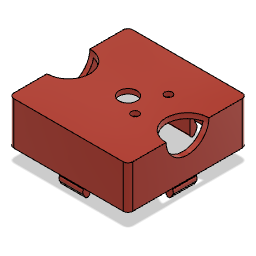
probatio_block_top_rotary_encoder_unthreaded_with_breakout_board_v2 (Autodesk Fusion 360 design; units mm, degrees)
Autodesk Fusion 360 part; units mm, degrees
note: some values were not read from the file. Chosen so that the rebuilt part matches the saved one: which face or edge a step refers to. Set by a fixed rule: which sketch regions a step uses.
ref_plane "WorkPlane1" through (0, 0, 56) normal (0, 0, 1) x (1, 0, 0)
sketch "top" plane through (0, 0, 56) normal (0, 0, 1) x (1, 0, 0)
  line L0 (25, -25) -> (-25, -25)
  line L1 (-25, -25) -> (-25, 25)
  line L2 (-25, 25) -> (25, 25)
  line L3 (25, 25) -> (25, -25)
  line L4 (25, -25) -> (-25, 25) construction
  line L5 (-25, -25) -> (25, 25) construction
  dimension "d12" = 50
  dimension "d13" = 50
  constraint perpendicular L0 L1
  constraint parallel L0 L2
  constraint parallel L1 L3
  constraint horizontal L0
  constraint coincident L4 origin
  constraint coincident L5 origin
  measures "d12" distance of L0.end L1.end
  measures "d13" distance of L1.end L2.end
extrude "Extrude1" add sketch "top" against normal blind 18 makes body 1
fillet "Fillet1" radius 2 4 edges at (-25, 25, 47) (25, 25, 47) (25, -25, 47) (-25, -25, 47) on bodies 1
shell "Shell1" thickness 2 removed faces 1 at (8.3333, -7.6667, 38) on bodies 1
sketch "handle" plane through (25, 0, 0) normal (1, 0, 0) x (0, 0, -1)
  line L0 (-38, -23) -> (-38, 23)
  line L1 (-56, 23) -> (-56, -23)
  line L2 (-56, 23) -> (-56, -23)
  circle A0 centre (-56, 0) radius 7
  line L3 (-56, -23) -> (-38, -23)
  line L4 (-38, 23) -> (-56, 23)
  line L5 (-38, 23) -> (-38, -23)
  circle A1 centre (-56, 0) radius 9
  dimension "d95" = 14
  dimension "d159" = 2
  constraint midpoint L1 A0.centre
  constraint concentric A0 A1
  measures "d95" diameter of A0
  measures "d159" distance of A0 A1
revolve "Revolve1" cut sketch "handle" angle 90 about axis through (25, 23, 56) along (0, 1, 0) contours L1 L2 A0 picked at (-50.399, -0.5675) bodies 1
revolve "Revolve2" cut sketch "handle" angle 90 about axis through (25, 23, 56) along (0, 1, 0) contours L1 L2 A0 A1 picked at (-54.0705, -8.0868) bodies 1
mirror "Mirror9" about plane through (0, 0, 0) normal (1, 0, 0) of "Revolve1", "Revolve2"
sketch "customisable" plane through (0, 0, 56) normal (0, 0, 1) x (1, 0, 0)
  line L0 (-25, -9) -> (-25, -23)
  line L1 (-23, -25) -> (23, -25)
  line L2 (23, 25) -> (-23, 25)
  line L3 (0.05, 0.05) -> (-0.05, 0.05)
  line L4 (-0.05, 0.05) -> (-0.05, -0.05)
  line L5 (-0.05, -0.05) -> (0.05, -0.05)
  line L6 (0.05, -0.05) -> (0.05, 0.05)
  line L7 (0.05, 0.05) -> (-0.05, -0.05) construction
  line L8 (-0.05, 0.05) -> (0.05, -0.05) construction
  arc A0 (-25, -23) -> (-23, -25) centre (-23, -23) ccw
  arc A1 (23, -25) -> (25, -23) centre (23, -23) ccw
  line L9 (25, -23) -> (25, -9)
  arc A2 (25, 23) -> (23, 25) centre (23, 23) ccw
  arc A3 (-23, 25) -> (-25, 23) centre (-23, 23) ccw
  arc A4 (-25, -9) -> (-25, 9) centre (-25, 0) ccw
  arc A5 (25, 9) -> (25, -9) centre (25, 0) ccw
  line L10 (25, 9) -> (25, 23)
  line L11 (-25, 23) -> (-25, 9)
  dimension "d104" = 0.1
  dimension "d105" = 0.1
  constraint perpendicular L3 L4
  constraint parallel L3 L5
  constraint parallel L4 L6
  constraint horizontal L3
  constraint coincident L7 origin
  constraint coincident L8 origin
  measures "d104" distance of L3.start L3.end
  measures "d105" distance of L3.start L5.end
extrude "Extrude4" [suppressed]
sketch "snap" plane through (0, 0, 0) normal (1, 0, 0) x (0, 0, -1)
  line L0 (-28, -48) -> (0, -48)
  line L1 (0, -48) -> (0, 48)
  line L2 (0, 48) -> (-28, 48)
  line L3 (-28, 48) -> (-28, -48)
  arc A0 (-38, 23) -> (-37.2488, 23.2186) centre (-38, 24.4) ccw
  line L4 (-37.2488, 23.2186) -> (-36.3595, 23.7321)
  arc A1 (-34.3595, 23.7321) -> (-36.3595, 23.7321) centre (-35.3595, 22) ccw
  line L5 (-34.3595, 23.7321) -> (-33.0915, 23)
  arc A2 (-32.5957, 22.2256) -> (-33.0915, 23) centre (-33.5915, 22.134) ccw
  line L6 (-32.5957, 22.2256) -> (-32.5834, 22.0917)
  arc A3 (-33.5792, 21) -> (-32.5834, 22.0917) centre (-33.5792, 22) ccw
  line L7 (-33.5792, 21) -> (-40.9732, 21)
  arc A4 (-42.0232, 21.2813) -> (-40.9732, 21) centre (-40.9732, 23.1) ccw
  line L8 (-42.0232, 21.2813) -> (-45, 23)
  line L9 (-45, 23) -> (-38, 23)
  line L10 (-54, 23) -> (-38, 23)
  line L11 (-38, 23) -> (-54, 23)
  dimension "d140" = 2
  dimension "d141" = 1
  dimension "d143" = 2.1
  dimension "d144" = 1.4
  dimension "d145" = 2
  dimension "d146" = 30
  dimension "d147" = 150
  dimension "d148" = 30
  dimension "d149" = 1
  dimension "d150" = 7
  constraint tangent A0 L9
  constraint horizontal L9
  constraint horizontal L7
  constraint tangent L4 A1
  constraint tangent A1 L5
  constraint tangent L5 A2
  constraint tangent A3 L7
  constraint tangent L7 A4
  constraint tangent A4 L8
  constraint tangent A2 L6
  constraint tangent L6 A3
  constraint horizontal A0.start L5.end
  constraint equal A2 A3
  constraint coincident A0.start L9.end
  measures "d140" radius of A1
  measures "d141" radius of A2
  measures "d143" radius of A4
  measures "d144" radius of A0
  measures "d145" distance of A0.start L7
  measures "d146" angle of L8 L9
  measures "d147" angle of L4 L9
  measures "d148" angle of L5 L9
  measures "d149" vertical distance of A0.start A1.centre
  measures "d150" distance of A0.start L8.end
extrude "Extrude5" add sketch "snap" along normal mid plane 10 separate body contours A0 L4 A1 L5 A2 L6 A3 L7 A4 L8 L9 L10 L11 makes body 2
mirror "Mirror6" about plane through (0, 0, 0) normal (0, 1, 0) of "Extrude5" makes body 3
copy_body "CopyPasteBodies2" bodies 2 makes body 4
move_body "Move4" bodies 4 to x (0, -1, 0) y (1, 0, 0) z (0, 0, 1) at (-26, 16, 0)
move_body "Move5" bodies 4 to x (1, 0, 0) y (0, 1, 0) z (0, 0, 1) at (26, -16, 0)
mirror "Mirror7" about plane through (0, 0, 0) normal (1, 0, 0) of bodies 4 makes body 5
combine "Combine2" operation add target body 1 tool bodies 2 3 5 4
move_body "Move6" bodies 1 to x (1, 0, 0) y (0, 0, -1) z (0, 1, 0) at (0, -57.5792, 7.5792)
ref_plane "WorkPlane2" through (0, -10.5792, 7.5792) normal (0, 0, 1) x (-1, 0, 0)
sketch "Sketch7" plane through (0, -1.5792, 0) normal (0, 1, 0) x (-1, 0, 0)
  arc A0 (25, 16.5792) -> (25, -1.4208) centre (25, 7.5792) ccw
  line L0 (25, 16.5792) -> (25, 30.5792)
  arc A1 (25, 30.5792) -> (23, 32.5792) centre (23, 30.5792) ccw
  line L1 (23, 32.5792) -> (-23, 32.5792)
  arc A2 (-23, 32.5792) -> (-25, 30.5792) centre (-23, 30.5792) ccw
  line L2 (-25, 30.5792) -> (-25, 16.5792)
  arc A3 (-25, -1.4208) -> (-25, 16.5792) centre (-25, 7.5792) ccw
  line L3 (-25, -1.4208) -> (-25, -15.4208)
  arc A4 (-25, -15.4208) -> (-23, -17.4208) centre (-23, -15.4208) ccw
  line L4 (-23, -17.4208) -> (23, -17.4208)
  arc A5 (23, -17.4208) -> (25, -15.4208) centre (23, -15.4208) ccw
  line L5 (25, -15.4208) -> (25, -1.4208)
  circle A6 centre (0, -3) radius 8 construction
  circle A7 centre (0, 18.1584) radius 8 construction
  line L6 (23, -15.4208) -> (-23, 30.5792) construction
  line L7 (-23, -15.4208) -> (23, 30.5792) construction
  circle A8 centre (0, 7.5792) radius 3.75 construction
  dimension "d16" = 16
  dimension "d18" = 16
  dimension "d21" = 7.5
  constraint coincident A5.centre L6.start
  constraint coincident A2.centre L6.end
  constraint coincident A4.centre L7.start
  constraint coincident A1.centre L7.end
  constraint midpoint L7 A8.centre
  measures "d16" diameter of A6
  measures "d18" diameter of A7
  measures "d21" diameter of A8
sketch "Sketch8" plane through (0, -1.5792, 0) normal (0, 1, 0) x (-1, 0, 0)
  circle A0 centre (0, 7.5792) radius 3.75
  point P0 (0, 7.5792)
  dimension "d23" = 7.5
  constraint coincident P0 A0.centre
  measures "d23" diameter of A0
extrude "Extrude10" cut sketch "Sketch8" against normal blind 13 bodies 1
sketch "Sketch9" plane through (0, -3.5792, 0) normal (0, -1, 0) x (1, 0, 0)
  circle A0 centre (0, 7.5792) radius 3.75
  arc A1 (-23, -0.9648) -> (-23, 16.1232) centre (-25, 7.5792) ccw
  line L0 (-23, -0.9648) -> (-23, -15.4208)
  line L1 (-23, -15.4208) -> (23, -15.4208)
  line L2 (23, -15.4208) -> (23, -0.9648)
  arc A2 (23, 16.1232) -> (23, -0.9648) centre (25, 7.5792) ccw
  line L3 (23, 16.1232) -> (23, 30.5792)
  line L4 (23, 30.5792) -> (-23, 30.5792)
  line L5 (-23, 30.5792) -> (-23, 16.1232)
  line L6 (0, 0) -> (0, 22.5652)
  line L7 (8, -0.5623) -> (8, 26.3303)
  circle A3 centre (8, 12.5792) radius 1.6
  circle A4 centre (8, -1.4208) radius 1.6
  line L8 (0, 7.5792) -> (8, 7.5792)
  line L9 (-7.1826, 15.5792) -> (12.1893, 15.5792)
  line L10 (8, -1.4208) -> (-11.6647, -1.4208)
  line L11 (-4, -5.8055) -> (-4, 16.681)
  circle A5 centre (-4, -1.4208) radius 2
  circle A6 centre (-4, 15.5792) radius 2
  dimension "d26" = 8
  dimension "d27" = 3.2
  dimension "d28" = 3.2
  dimension "d29" = 9
  dimension "d30" = 5
  dimension "d37" = 12
  dimension "d38" = 4
  dimension "d39" = 17
  dimension "d40" = 4
  constraint coincident L6.start origin
  constraint vertical L6
  constraint vertical L7
  constraint coincident L7 A3.centre
  constraint coincident L7 A4.centre
  constraint coincident A0.centre L8.start
  constraint coincident L7 L8.end
  constraint perpendicular L7 L8
  constraint perpendicular L7 L9
  constraint coincident A4.centre L10.start
  constraint horizontal L10
  constraint vertical L11
  constraint coincident L11 A5.centre
  constraint coincident L10 A5.centre
  constraint coincident L11 A6.centre
  constraint coincident L9 A6.centre
  measures "d26" distance of L6 L7
  measures "d27" diameter of A3
  measures "d28" diameter of A4
  measures "d29" distance of A4.centre L8.end
  measures "d30" distance of A3.centre L8
  measures "d37" distance of L7 L11
  measures "d38" diameter of A5
  measures "d39" distance of L9 L10
  measures "d40" diameter of A6
extrude "Extrude13" cut sketch "Sketch9" against normal blind 15 contours A4 | L7 A3 | L7 A3 bodies 1
extrude "Extrude11" [suppressed]
sketch "Sketch10" plane through (0, -10.5792, 0) normal (0, -1, 0) x (1, 0, 0)
  circle A0 centre (8, -1.4208) radius 2.25
  circle A1 centre (8, 12.5792) radius 2.25
  circle A2 centre (8, 12.5792) radius 1.25
  circle A3 centre (8, -1.4208) radius 1.25
  dimension "d33" = 2.5
  dimension "d34" = 2.5
  constraint concentric A1 A2
  constraint concentric A0 A3
  measures "d33" diameter of A2
  measures "d34" diameter of A3
extrude "Extrude12" [suppressed]
ref_plane "WorkPlane4" through (0, -10.5792, 7.5792) normal (-1, 0, 0) x (0, 0, -1)
equation "d11 = height"
equation "d12 = ( length_blocks * 50 ) * 1 mm"
equation "d13 = ( width_blocks * 50 ) * 1 mm"
equation "d14 = -height / 2 + 10 mm"
equation "d57 = thickness"
equation "d104 = customisable_rectangle"
equation "d105 = d104"
equation "height = 56 mm"
equation "customisable_rectangle = 0.1 mm"
equation "width_blocks = 1"
equation "length_blocks = 1"
equation "thickness = 2 mm"
equation "dual_holes = 16 mm"
equation "d16 = dual_holes"
equation "d18 = dual_holes"
equation "centered_hole = 14 mm"
named bodies: "top", "snap1", "snap2", "snap3", "snap4"
